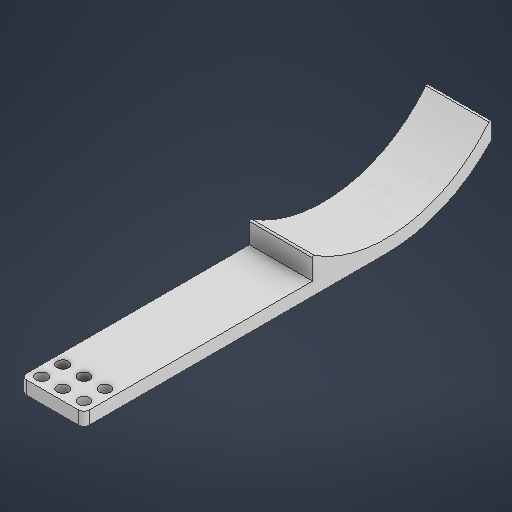
# Autodesk Inventor part: Launcher_Arm_V1
Saved by Autodesk Inventor 2026.1 (Build 301233020, 233B)
## iProperties
Created: 2025-11-02
Part Number: Launcher_Arm_V1
Material: Generic
Document SubType Name: Modeling
Designer: Asus
Density: 1 g/cm^3
Appearance: Default
Author: Asus
Autodesk Inventor part; units mm, degrees
ref_plane "YZ Plane" through (0, 0, 0) normal (1, 0, 0) x (0, 1, 0)
ref_plane "XZ Plane" through (0, 0, 0) normal (0, 1, 0) x (-1, 0, 0)
ref_plane "XY Plane" through (0, 0, 0) normal (0, 0, 1) x (1, 0, 0)
sketch "Sketch1" plane through (0, 0, 0) normal (0, 1, 0) x (-1, 0, 0)
  line L0 (-10, 77.5) -> (10, 77.5)
  line L1 (12, 75.5) -> (12, -77.5)
  line L2 (12, -77.5) -> (-12, -77.5)
  line L3 (-12, -77.5) -> (-12, 75.5)
  line L4 (-12, 77.5) -> (12, -77.5) construction
  line L5 (12, 77.5) -> (-12, -77.5) construction
  arc A0 (12, 75.5) -> (10, 77.5) centre (10, 75.5) ccw
  arc A1 (-10, 77.5) -> (-12, 75.5) centre (-10, 75.5) ccw
  circle A2 centre (8, 73.5) radius 2.2
  circle A3 centre (0, 73.5) radius 2.2
  circle A4 centre (-8, 73.5) radius 2.2
  circle A5 centre (8, 65.5) radius 2.2
  circle A6 centre (0, 65.5) radius 2.2
  circle A7 centre (-8, 65.5) radius 2.2
  point P0 (0, 0)
  dimension "d0" = 24
  dimension "d1" = 155
  dimension "d2" = 2
  dimension "d3" = 4.4
  dimension "d4" = 4
  dimension "d5" = 4
  dimension "d8" = 8
  dimension "d11" = 8
  constraints: 12 end point, 8 centre point, 4 point on circle, 4 point on line, 4 tangent, 2 horizontal, 2 midpoint, 2 parallel, 1 equal radius, 1 perpendicular, 1 vertical, 10 other
  measures "d0" distance of L1.end L2.end
  measures "d1" distance of L5.start L1.end
  measures "d2" radius of A0
  measures "d3" diameter of A2
  measures "d4" distance from line of L1 A2.centre
  measures "d5" distance from line of L0 A2.centre
  measures "d8" distance of A2.centre A3.centre
  measures "d11" distance of A2.centre A5.centre
extrude "Extrusion1" add sketch "Sketch1" along normal blind 5
sketch "Sketch2" plane through (12, 0, 75.5) normal (1, 0, 0) x (0, 0, -1)
  arc A0 (113, 5) -> (152.1089, 23.8473) centre (113, 55) ccw
  line L0 (0, 5) -> (153, 5) projected
  line L1 (153, 5) -> (153, 23.5357)
  arc A1 (153, 23.5357) -> (152.1089, 23.8473) centre (152.5, 23.5357) ccw
  point P0 (75.5, 0)
  point P1 (153, 25)
  dimension "d16" = 100
  dimension "d17" = 40
  dimension "d18" = 0.5
  constraints: 5 point on circle, 3 tangent, 2 centre point, 2 end point, 2 point on line, 1 vertical
  measures "d16" diameter of A0
  measures "d17" distance from line of L1 A0.centre
  measures "d18" radius of A1
extrude "Extrusion2" add sketch "Sketch2" against normal blind 24
sketch "Sketch3" plane through (12, 0, 75.5) normal (1, 0, 0) x (0, 0, -1)
  line L0 (0, 0) -> (153, 0) projected
  arc A0 (113, 5) -> (152.1089, 23.8473) centre (113, 55) ccw projected
  line L1 (0, 5) -> (113, 5) projected
  arc A1 (113, 0) -> (152.8624, 17.1055) centre (113, 55) ccw
  line L2 (153, 0) -> (153, 23.5357) projected
  line L3 (153, 17.2508) -> (153, 0)
  line L4 (153, 0) -> (113, 0)
  arc A2 (152.8624, 17.1055) -> (153, 17.45) centre (152.5, 17.45) ccw
  point P0 (150, 0)
  dimension "d27" = 1
  dimension "d28" = 17.2508
  constraints: 4 end point, 4 point on circle, 3 tangent, 2 centre point, 2 point on line, 1 coincident, 1 vertical
  measures "d27" diameter of A2
  measures "d28" distance of L0.end L3.start
extrude "Extrusion3" cut sketch "Sketch3" against normal blind 24
sketch "Sketch4" plane through (12, 0, 75.5) normal (1, 0, 0) x (0, 0, -1)
  arc A0 (85.7723, 13.0637) -> (113, 5) centre (113, 55) ccw
  line L0 (0, 5) -> (113, 5) projected
  line L1 (153, 17.45) -> (153, 23.5357) projected
  line L2 (85, 5) -> (85, 12.6444)
  arc A1 (85.7723, 13.0637) -> (85, 12.6444) centre (85.5, 12.6444) ccw
  point P0 (75.5, 0)
  point P1 (85, 13.5754)
  dimension "d31" = 0.5
  constraints: 5 point on circle, 3 end point, 3 tangent, 2 centre point, 2 point on line, 1 perpendicular
  measures "d31" radius of A1
extrude "Extrusion4" add sketch "Sketch4" against normal blind 24
body "Solid1"
